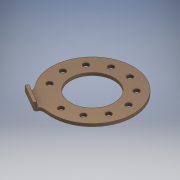
# Autodesk Inventor part: SŁONECZKO MAŁE Z BLOKADĄ
Saved by Autodesk Inventor 2017 SP1 (Build 210196100, 196)
## iProperties
Created: 2021-01-30
Part Number: SŁONECZKO MAŁE Z BLOKADĄ
Material: Stal
Document SubType Name: Modeling
Designer: Napoleon
Mass: 0.497645 g
Surface Area: 3.0679 cm^2
Volume: 0.0633943 cm^3
Density: 7.85 g/cm^3
Appearance: Anodowany - brązowy
Author: Napoleon
Autodesk Inventor part; units mm, degrees
ref_plane "YZ Plane" through (0, 0, 0) normal (1, 0, 0) x (0, 1, 0)
ref_plane "XZ Plane" through (0, 0, 0) normal (0, 1, 0) x (-1, 0, 0)
ref_plane "XY Plane" through (0, 0, 0) normal (0, 0, 1) x (1, 0, 0)
sketch "Szkic1" plane through (0, 0, 0) normal (0, 0, 1) x (1, 0, 0)
  arc A0 (-0.9737, -7.4365) -> (-5.9534, -4.5615) centre (0, 0) ccw
  circle A1 centre (0, 0) radius 4
  circle A2 centre (0, -5.75) radius 0.5
  circle A3 centre (3.1597, -4.8041) radius 0.5
  circle A4 centre (5.2797, -2.2775) radius 0.5
  circle A5 centre (5.6626, 0.9985) radius 0.5
  circle A6 centre (4.1824, 3.9459) radius 0.5
  circle A7 centre (1.326, 5.595) radius 0.5
  circle A8 centre (-1.9666, 5.4032) radius 0.5
  circle A9 centre (-4.6122, 3.4337) radius 0.5
  circle A10 centre (-5.7403, 0.3343) radius 0.5
  circle A11 centre (-4.9796, -2.875) radius 0.5
  arc A12 (-5.4821, -5.4952) -> (-5.9534, -4.5615) centre (-8.3548, -6.3596) ccw
  arc A13 (-0.9737, -7.4365) -> (-2.0179, -7.4952) centre (-1.3301, -10.4153) ccw
  line L0 (-5.4821, -5.4952) -> (-5.9821, -6.3612)
  line L1 (-2.0179, -7.4952) -> (-2.5179, -8.3612)
  line L2 (-2.5179, -8.3612) -> (-5.9821, -6.3612)
  dimension "d0" = 15
  dimension "d1" = 8
  dimension "d2" = 1
  dimension "d5" = 300
  constraints: 14 centre point, 6 end point, 6 point on circle, 2 coincident, 1 perpendicular, 19 other
  measures "d0" diameter of A0
  measures "d1" diameter of A1
  measures "d2" diameter of A2
extrude "Wyciągnięcie proste1" add sketch "Szkic1" along normal mid plane 0.5
sketch "Szkic2" plane through (0, 0, 0.25) normal (0, 0, 1) x (1, 0, 0)
  line L0 (-5.9821, -6.3612) -> (-2.5179, -8.3612)
  line L1 (-2.2679, -7.9282) -> (-5.7321, -5.9282)
  line L2 (-5.7321, -5.9282) -> (-5.9821, -6.3612)
  line L3 (-2.2679, -7.9282) -> (-2.5179, -8.3612)
  constraints: 8 end point
extrude "Wyciągnięcie proste2" add sketch "Szkic2" along normal blind 1
fillet "Zaokrąglenie1" radius 0.5 1 edges at (-4.25, -7.3612, -0.25)
fillet "Zaokrąglenie2" radius 0.25 1 edges at (-4, -6.9282, 0.25)
